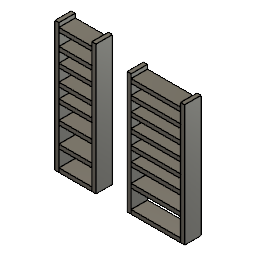
Shelves v2 (Autodesk Fusion 360 design; units mm, degrees)
Autodesk Fusion 360 part; units mm, degrees
note: some values were not read from the file. Chosen so that the rebuilt part matches the saved one: which bodies a step acts on.
sketch "Sketch2" plane through (0, 0, 0) normal (0, 1, 0) x (1, 0, 0)
  line L0 (0, 0) -> (2, 0)
  line L1 (2, 0) -> (2, -8)
  line L2 (2, -8) -> (0, -8)
  line L3 (0, -8) -> (0, 0)
  line L4 (2, 0) -> (18, 0)
  line L5 (18, 0) -> (20, 0)
  line L6 (20, 0) -> (20, -8)
  line L7 (20, -8) -> (18, -8)
  line L8 (18, -8) -> (18, 0)
  dimension "d5" = 8
  dimension "d6" = 2
  dimension "d7" = 16
  dimension "d8" = 2
  constraint horizontal L0
  constraint vertical L1
  constraint horizontal L2
  constraint vertical L3
  constraint coincident L0.start L3.end
  constraint perpendicular L1 L4
  constraint horizontal L5
  constraint vertical L6
  constraint horizontal L7
  constraint vertical L8
  measures "d5" distance of L0.start L2.end
  measures "d6" distance of L0.start L0.end
  measures "d7" distance of L0.end L4.end
  measures "d8" distance of L4.end L5.end
extrude "Extrude2" add sketch "Sketch2" along normal blind 60 makes body 1 at (20, 20, 2.6667) makes body 2 at (2, 20, 2.6667)
sketch "Sketch3" plane through (0, 0, 0) normal (0, 1, 0) x (1, 0, 0)
  line L0 (2, 0) -> (18, 0)
  line L1 (18, 0) -> (18, -8)
  line L2 (18, -8) -> (2, -8)
  line L3 (2, -8) -> (2, 0)
  constraint horizontal L0
  constraint vertical L1
  constraint horizontal L2
  constraint vertical L3
extrude "Extrude3" add sketch "Sketch3" along normal blind 60 separate body makes body 3
sketch "Sketch4" plane through (0, 0, 8) normal (0, 0, 1) x (1, 0, 0)
  line L0 (2, 0) -> (18, 0)
  line L1 (18, 0) -> (18, 60)
  line L2 (18, 60) -> (2, 60)
  line L3 (2, 60) -> (2, 0)
  line L4 (2, 0) -> (18, 0)
  line L5 (18, 0) -> (18, 2)
  line L6 (18, 2) -> (2, 2)
  line L7 (2, 2) -> (2, 0)
  line L8 (18, 2) -> (2, 2)
  line L9 (2, 2) -> (2, 10)
  line L10 (2, 10) -> (18, 10)
  line L11 (18, 10) -> (18, 2)
  line L12 (2, 10) -> (18, 10)
  line L13 (18, 10) -> (18, 12)
  line L14 (18, 12) -> (2, 12)
  line L15 (2, 12) -> (2, 10)
  line L16 (18, 12) -> (2, 12)
  line L17 (2, 12) -> (2, 20)
  line L18 (2, 20) -> (18, 20)
  line L19 (18, 20) -> (18, 12)
  line L20 (2, 20) -> (18, 20)
  line L21 (18, 20) -> (18, 22)
  line L22 (18, 22) -> (2, 22)
  line L23 (2, 22) -> (2, 20)
  line L24 (18, 22) -> (2, 22)
  line L25 (2, 22) -> (2, 29)
  line L26 (2, 29) -> (18, 29)
  line L27 (18, 29) -> (18, 22)
  line L28 (2, 29) -> (18, 29)
  line L29 (18, 29) -> (18, 31)
  line L30 (18, 31) -> (2, 31)
  line L31 (2, 31) -> (2, 29)
  line L32 (18, 31) -> (2, 31)
  line L33 (2, 31) -> (2, 36)
  line L34 (2, 36) -> (18, 36)
  line L35 (18, 36) -> (18, 31)
  line L36 (2, 36) -> (18, 36)
  line L37 (18, 36) -> (18, 38)
  line L38 (18, 38) -> (2, 38)
  line L39 (2, 38) -> (2, 36)
  line L40 (18, 38) -> (2, 38)
  line L41 (2, 38) -> (2, 44)
  line L42 (2, 44) -> (18, 44)
  line L43 (18, 44) -> (18, 38)
  line L44 (2, 44) -> (18, 44)
  line L45 (18, 44) -> (18, 46)
  line L46 (18, 46) -> (2, 46)
  line L47 (2, 46) -> (2, 44)
  line L48 (18, 46) -> (2, 46)
  line L49 (2, 46) -> (2, 51)
  line L50 (2, 51) -> (18, 51)
  line L51 (18, 51) -> (18, 46)
  line L52 (2, 51) -> (18, 51)
  line L53 (18, 51) -> (18, 53)
  line L54 (18, 53) -> (2, 53)
  line L55 (2, 53) -> (2, 51)
  line L56 (2, 53) -> (18, 53)
  line L57 (18, 53) -> (18, 59)
  line L58 (18, 59) -> (2, 59)
  line L59 (2, 59) -> (2, 53)
  dimension "d13" = 2
  dimension "d14" = 8
  dimension "d15" = 2
  dimension "d16" = 8
  dimension "d17" = 2
  dimension "d18" = 7
  dimension "d19" = 2
  dimension "d20" = 5
  dimension "d21" = 2
  dimension "d22" = 6
  dimension "d23" = 2
  dimension "d24" = 5
  dimension "d26" = 2
  dimension "d27" = 6
  constraint horizontal L4
  constraint vertical L5
  constraint horizontal L6
  constraint vertical L7
  constraint coincident L0.start L3.end
  constraint horizontal L8
  constraint vertical L9
  constraint horizontal L10
  constraint vertical L11
  constraint horizontal L12
  constraint vertical L13
  constraint horizontal L14
  constraint vertical L15
  constraint horizontal L16
  constraint vertical L17
  constraint horizontal L18
  constraint vertical L19
  constraint horizontal L20
  constraint vertical L21
  constraint horizontal L22
  constraint vertical L23
  constraint horizontal L24
  constraint vertical L25
  constraint horizontal L26
  constraint vertical L27
  constraint horizontal L28
  constraint vertical L29
  constraint horizontal L30
  constraint vertical L31
  constraint horizontal L32
  constraint vertical L33
  constraint horizontal L34
  constraint vertical L35
  constraint horizontal L36
  constraint vertical L37
  constraint horizontal L38
  constraint vertical L39
  constraint horizontal L40
  constraint vertical L41
  constraint horizontal L42
  constraint vertical L43
  constraint horizontal L44
  constraint vertical L45
  constraint horizontal L46
  constraint vertical L47
  constraint horizontal L48
  constraint vertical L49
  constraint horizontal L50
  constraint vertical L51
  constraint horizontal L52
  constraint vertical L53
  constraint horizontal L54
  constraint vertical L55
  constraint horizontal L56
  constraint vertical L57
  constraint horizontal L58
  constraint vertical L59
  measures "d13" distance of L0.start L6.end
  measures "d14" distance of L5.end L10.end
  measures "d15" distance of L9.end L14.end
  measures "d16" distance of L13.end L18.end
  measures "d17" distance of L17.end L22.end
  measures "d18" distance of L21.end L26.end
  measures "d19" distance of L25.end L30.end
  measures "d20" distance of L29.end L34.end
  measures "d21" distance of L33.end L38.end
  measures "d22" distance of L37.end L42.end
  measures "d23" distance of L41.end L46.end
  measures "d24" distance of L45.end L50.end
  measures "d26" distance of L49.end L54.end
  measures "d27" distance of L54.end L58.end
extrude "Extrude4" cut sketch "Sketch4" against normal blind 34 contours L1 L3 L6 L8 L9 L10 L11 L12 | L1 L3 L14 L16 L17 L18 L19 L20 | L1 L3 L22 L24 L25 L26 L27 L28 | L1 L3 L30 L32 L33 L34 L35 L36 | L1 L3 L38 L40 L41 L42 L43 L44 | L1 L3 L46 L48 L49 L50 L51 L52 | L1 L3 L54 L56 L57 L58 L59 bodies 3 makes body 4 at (7.3333, 44, 5.3333) makes body 5 at (7.3333, 10, 5.3333) makes body 6 at (7.3333, 36, 5.3333) makes body 7 at (12.6667, 51, 2.6667) makes body 8 at (7.3333, 60, 2.6667) makes body 9 at (7.3333, 20, 5.3333) makes body 10 at (7.3333, 0, 2.6667)
extrude "Extrude5" add 1 faces at (7.3333, 60, 2.6667) along direction (0, 1, 0) blind 1 on bodies 8 bodies 8
extrude "Extrude6" add 2 faces at (0.6667, 60, 2.6667) (18.6667, 60, 2.6667) along direction (0, 1, 0) blind 1 on bodies 1 2 bodies 2 1 3 4 5 6 7 10
sketch "Sketch5" plane through (0, 0, 0) normal (0, 1, 0) x (1, 0, 0)
  line L0 (35, 0) -> (37, 0)
  line L1 (37, 0) -> (37, -8)
  line L2 (37, -8) -> (35, -8)
  line L3 (35, -8) -> (35, 0)
  line L4 (37, 0) -> (61, 0)
  line L5 (61, 0) -> (61, -8)
  line L6 (61, -8) -> (37, -8)
  line L7 (37, -8) -> (37, 0)
  line L8 (61, -8) -> (63, -8)
  line L9 (63, -8) -> (63, 0)
  line L10 (63, 0) -> (61, 0)
  line L11 (61, 0) -> (61, -8)
  dimension "d34" = 2
  dimension "d35" = 24
  dimension "d36" = 2
  constraint horizontal L0
  constraint vertical L1
  constraint horizontal L2
  constraint vertical L3
  constraint horizontal L4
  constraint vertical L5
  constraint horizontal L6
  constraint vertical L7
  constraint horizontal L8
  constraint vertical L9
  constraint horizontal L10
  constraint vertical L11
  measures "d34" distance of L0.start L0.end
  measures "d35" distance of L0.end L4.end
  measures "d36" distance of L5.end L8.end
extrude "Extrude7" add sketch "Sketch5" along normal blind 61 separate body contours L0 L1 L2 L3 L7 | L5 L8 L9 L10 L11 makes body 11 at (63, 20.3333, 5.3333) makes body 12 at (37, 20.3333, 2.6667)
sketch "Sketch6" plane through (0, 0, 0) normal (0, 1, 0) x (1, 0, 0)
  line L0 (37, 0) -> (61, 0)
  line L1 (61, 0) -> (61, -8)
  line L2 (61, -8) -> (37, -8)
  line L3 (37, -8) -> (37, 0)
  constraint horizontal L0
  constraint vertical L1
  constraint horizontal L2
  constraint vertical L3
extrude "Extrude8" add sketch "Sketch6" along normal blind 61 separate body makes body 13
sketch "Sketch7" plane through (0, 0, 8) normal (0, 0, 1) x (1, 0, 0)
  line L0 (37, 0) -> (61, 0)
  line L1 (61, 0) -> (61, 61)
  line L2 (61, 61) -> (37, 61)
  line L3 (37, 61) -> (37, 0)
  line L4 (37, 0) -> (61, 0)
  line L5 (61, 0) -> (61, 2)
  line L6 (61, 2) -> (37, 2)
  line L7 (37, 2) -> (37, 0)
  line L8 (61, 2) -> (37, 2)
  line L9 (37, 2) -> (37, 11)
  line L10 (37, 11) -> (61, 11)
  line L11 (61, 11) -> (61, 2)
  line L12 (37, 11) -> (61, 11)
  line L13 (61, 11) -> (61, 13)
  line L14 (61, 13) -> (37, 13)
  line L15 (37, 13) -> (37, 11)
  line L16 (61, 13) -> (37, 13)
  line L17 (37, 13) -> (37, 20)
  line L18 (37, 20) -> (61, 20)
  line L19 (61, 20) -> (61, 13)
  line L20 (37, 20) -> (61, 20)
  line L21 (61, 20) -> (61, 22)
  line L22 (61, 22) -> (37, 22)
  line L23 (37, 22) -> (37, 20)
  line L24 (61, 22) -> (37, 22)
  line L25 (37, 22) -> (37, 27)
  line L26 (37, 27) -> (61, 27)
  line L27 (61, 27) -> (61, 22)
  line L28 (37, 27) -> (61, 27)
  line L29 (61, 27) -> (61, 29)
  line L30 (61, 29) -> (37, 29)
  line L31 (37, 29) -> (37, 27)
  line L32 (61, 29) -> (37, 29)
  line L33 (37, 29) -> (37, 34)
  line L34 (37, 34) -> (61, 34)
  line L35 (61, 34) -> (61, 29)
  line L36 (37, 34) -> (61, 34)
  line L37 (61, 34) -> (61, 36)
  line L38 (61, 36) -> (37, 36)
  line L39 (37, 36) -> (37, 34)
  line L40 (61, 36) -> (37, 36)
  line L41 (37, 36) -> (37, 41)
  line L42 (37, 41) -> (61, 41)
  line L43 (61, 41) -> (61, 36)
  line L44 (37, 41) -> (61, 41)
  line L45 (61, 41) -> (61, 43)
  line L46 (61, 43) -> (37, 43)
  line L47 (37, 43) -> (37, 41)
  line L48 (61, 43) -> (37, 43)
  line L49 (37, 43) -> (37, 48)
  line L50 (37, 48) -> (61, 48)
  line L51 (61, 48) -> (61, 43)
  line L52 (37, 48) -> (61, 48)
  line L53 (61, 48) -> (61, 50)
  line L54 (61, 50) -> (37, 50)
  line L55 (37, 50) -> (37, 48)
  line L56 (61, 50) -> (37, 50)
  line L57 (37, 50) -> (37, 55)
  line L58 (37, 55) -> (61, 55)
  line L59 (61, 55) -> (61, 50)
  line L60 (37, 55) -> (61, 55)
  line L61 (61, 55) -> (61, 57)
  line L62 (61, 57) -> (37, 57)
  line L63 (37, 57) -> (37, 55)
  dimension "d41" = 2
  dimension "d42" = 9
  dimension "d43" = 2
  dimension "d44" = 7
  dimension "d45" = 2
  dimension "d46" = 5
  dimension "d47" = 2
  dimension "d48" = 5
  dimension "d49" = 2
  dimension "d50" = 5
  dimension "d51" = 2
  dimension "d52" = 5
  dimension "d53" = 2
  dimension "d54" = 5
  dimension "d55" = 2
  constraint horizontal L4
  constraint vertical L5
  constraint horizontal L6
  constraint vertical L7
  constraint coincident L0.start L3.end
  constraint horizontal L8
  constraint vertical L9
  constraint horizontal L10
  constraint vertical L11
  constraint horizontal L12
  constraint vertical L13
  constraint horizontal L14
  constraint vertical L15
  constraint horizontal L16
  constraint vertical L17
  constraint horizontal L18
  constraint vertical L19
  constraint horizontal L20
  constraint vertical L21
  constraint horizontal L22
  constraint vertical L23
  constraint horizontal L24
  constraint vertical L25
  constraint horizontal L26
  constraint vertical L27
  constraint horizontal L28
  constraint vertical L29
  constraint horizontal L30
  constraint vertical L31
  constraint horizontal L32
  constraint vertical L33
  constraint horizontal L34
  constraint vertical L35
  constraint horizontal L36
  constraint vertical L37
  constraint horizontal L38
  constraint vertical L39
  constraint horizontal L40
  constraint vertical L41
  constraint horizontal L42
  constraint vertical L43
  constraint horizontal L44
  constraint vertical L45
  constraint horizontal L46
  constraint vertical L47
  constraint horizontal L48
  constraint vertical L49
  constraint horizontal L50
  constraint vertical L51
  constraint horizontal L52
  constraint vertical L53
  constraint horizontal L54
  constraint vertical L55
  constraint horizontal L56
  constraint vertical L57
  constraint horizontal L58
  constraint vertical L59
  constraint horizontal L60
  constraint vertical L61
  constraint horizontal L62
  constraint vertical L63
  measures "d41" distance of L0.start L6.end
  measures "d42" distance of L5.end L10.end
  measures "d43" distance of L9.end L14.end
  measures "d44" distance of L13.end L18.end
  measures "d45" distance of L17.end L22.end
  measures "d46" distance of L21.end L26.end
  measures "d47" distance of L25.end L30.end
  measures "d48" distance of L29.end L34.end
  measures "d49" distance of L33.end L38.end
  measures "d50" distance of L37.end L42.end
  measures "d51" distance of L41.end L46.end
  measures "d52" distance of L45.end L50.end
  measures "d53" distance of L49.end L54.end
  measures "d54" distance of L53.end L58.end
  measures "d55" distance of L57.end L62.end
extrude "Extrude9" cut sketch "Sketch7" against normal blind 46 contours L1 L3 L6 L8 L9 L10 L11 L12 | L1 L3 L14 L16 L17 L18 L19 L20 | L1 L3 L22 L24 L25 L26 L27 L28 | L1 L3 L30 L32 L33 L34 L35 L36 | L1 L3 L38 L40 L41 L42 L43 L44 | L1 L3 L46 L48 L49 L50 L51 L52 | L1 L3 L54 L56 L57 L58 L59 L60 | L1 L2 L3 L62 bodies 13 makes body 14 at (45, 34, 2.6667) makes body 15 at (45, 11, 2.6667) makes body 16 at (45, 41, 2.6667) makes body 17 at (45, 55, 2.6667) makes body 18 at (45, 48, 2.6667) makes body 19 at (45, 20, 2.6667) makes body 20 at (45, 0, 5.3333)
extrude "Extrude10" add 2 faces at (0.6667, 61, 2.6667) (18.6667, 61, 2.6667) along direction (0, 1, 0) blind 2 on bodies 1 2 bodies 2 1 3 4 5 6 7 9 10
extrude "Extrude11" cut 2 faces at (35.6667, 61, 2.6667) (61.6667, 61, 2.6667) along direction (0, -1, 0) blind 2 on bodies 11 12 bodies 11 12
